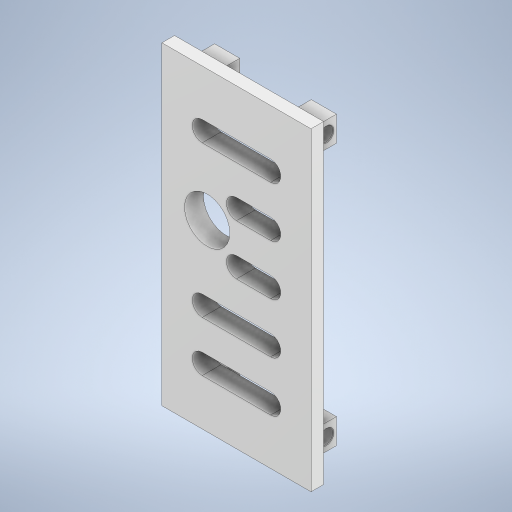
# Autodesk Inventor part: SENSOR_TOP
Saved by Autodesk Inventor 2023 (Build 270158000, 158)
## iProperties
Created: 2023-03-28
Part Number: SENSOR_TOP
Material: PC/ABS Plastic
Document SubType Name: Modeling
Designer: catsm
Density: 0.357273 g/cm^3
Appearance: Smooth - White
Author: catsm
Autodesk Inventor part; units mm, degrees
ref_plane "YZ Plane" through (0, 0, 0) normal (1, 0, 0) x (0, 1, 0)
ref_plane "XZ Plane" through (0, 0, 0) normal (0, 1, 0) x (-1, 0, 0)
ref_plane "XY Plane" through (0, 0, 0) normal (0, 0, 1) x (1, 0, 0)
sketch "Sketch1" plane through (0, 0, 0) normal (0, 0, 1) x (1, 0, 0)
  line L0 (-18.7833, 39.6114) -> (-18.7833, -39.6114) projected
  line L1 (-18.7833, -39.6114) -> (18.7833, -39.6114) projected
  line L2 (18.7833, -39.6114) -> (18.7833, 39.6114) projected
  line L3 (18.7833, 39.6114) -> (-18.7833, 39.6114) projected
  line L4 (-15.6083, 36.4364) -> (15.6083, 36.4364) projected
  line L5 (15.6083, 36.4364) -> (15.6083, -36.4364) projected
  line L6 (15.6083, -36.4364) -> (-15.6083, -36.4364) projected
  line L7 (-15.6083, -36.4364) -> (-15.6083, 36.4364) projected
  point P0 (0, 0)
extrude "Extrusion1" add sketch "Sketch1" along normal blind 3.175 contours L3 L2 L1 L0 | L4 L5 L6 L7
sketch "Sketch2" plane through (0, 0, 0) normal (0, 0, -1) x (-1, 0, 0)
  line L0 (-15.6083, -36.4364) -> (15.6083, -36.4364) projected
  line L1 (-15.6083, 36.4364) -> (-15.6083, -36.4364) projected
  line L2 (15.6083, 36.4364) -> (-15.6083, 36.4364) projected
  line L3 (15.6083, -36.4364) -> (15.6083, 36.4364) projected
  line L4 (-15.3543, 36.1824) -> (-15.3543, -36.1824)
  line L5 (-15.3543, -36.1824) -> (15.3543, -36.1824)
  line L6 (15.3543, -36.1824) -> (15.3543, 36.1824)
  line L7 (15.3543, 36.1824) -> (-15.3543, 36.1824)
  point P0 (0, 0)
  dimension "d2" = 0.254
  constraints: 8 end point, 3 other
  measures "d2" distance between parallel lines of L2 L7
extrude "Extrusion2" add sketch "Sketch2" along normal blind 1.5875 contours L7 L6 L5 L4
sketch "Sketch3" plane through (0, 0, -1.5875) normal (0, 0, -1) x (-1, 0, 0)
  line L0 (-15.3543, 36.1824) -> (-15.3543, -36.1824) projected
  line L1 (-15.3543, 36.1824) -> (-9.0043, 36.1824)
  line L2 (-9.0043, 36.1824) -> (-9.0043, 29.8324)
  line L3 (-9.0043, 29.8324) -> (-15.3543, 29.8324)
  line L4 (-15.3543, 29.8324) -> (-15.3543, 36.1824)
  line L5 (15.3543, 36.1824) -> (-15.3543, 36.1824) projected
  line L6 (15.3543, 36.1824) -> (9.0043, 36.1824)
  line L7 (9.0043, 36.1824) -> (9.0043, 29.8324)
  line L8 (9.0043, 29.8324) -> (15.3543, 29.8324)
  line L9 (15.3543, 29.8324) -> (15.3543, 36.1824)
  line L10 (-15.3543, -36.1824) -> (15.3543, -36.1824) projected
  line L11 (-15.3543, -36.1824) -> (-9.0043, -36.1824)
  line L12 (-9.0043, -36.1824) -> (-9.0043, -29.8324)
  line L13 (-9.0043, -29.8324) -> (-15.3543, -29.8324)
  line L14 (-15.3543, -29.8324) -> (-15.3543, -36.1824)
  line L15 (15.3543, 36.1824) -> (15.3543, -36.1824) projected
  line L16 (15.3543, -36.1824) -> (9.0043, -36.1824)
  line L17 (9.0043, -36.1824) -> (9.0043, -29.8324)
  line L18 (9.0043, -29.8324) -> (15.3543, -29.8324)
  line L19 (15.3543, -29.8324) -> (15.3543, -36.1824)
  point P0 (0, 0)
  dimension "d5" = 6.35
  dimension "d6" = 6.35
  dimension "d7" = 6.35
  dimension "d8" = 6.35
  dimension "d9" = 6.35
  dimension "d10" = 6.35
  dimension "d11" = 6.35
  dimension "d12" = 6.35
  constraints: 32 end point, 8 parallel, 4 horizontal, 4 perpendicular
  measures "d5" distance of L2.end L3.end
  measures "d6" distance of L1.end L2.end
  measures "d7" distance of L8.end L7.end
  measures "d8" distance of L7.end L6.end
  measures "d9" distance of L13.end L12.end
  measures "d10" distance of L12.end L11.end
  measures "d11" distance of L17.end L18.end
  measures "d12" distance of L16.end L17.end
extrude "Extrusion3" add sketch "Sketch3" along normal blind 5.08 contours L1 L2 L3 L0 | L13 L12 L10 L0 | L5 L9 L8 L7 | L17 L18 L15 L10
sketch "Sketch4" plane through (15.3543, -36.1824, 0) normal (1, 0, 0) x (0, 0, -1)
  line L0 (6.6675, 66.0147) -> (6.6675, 72.3647) projected
  line L1 (0, 72.3647) -> (0, 0) projected
  line L2 (6.6675, 0) -> (6.6675, 6.35) projected
  line L3 (1.5875, 66.0147) -> (1.5875, 6.35) projected
  line L4 (0, 72.3647) -> (6.6675, 72.3647) projected
  line L5 (1.5875, 6.35) -> (6.6675, 6.35) projected
  line L6 (6.6675, 6.35) -> (6.6675, 0) projected
  line L7 (1.5875, 6.35) -> (6.6675, 0)
  line L8 (1.5875, 66.0147) -> (6.6675, 72.3647)
  point P0 (0, 36.1824)
  point P1 (4.1275, 3.175)
  point P2 (4.1275, 69.1897)
  point P3 (4.1275, 3.175)
  point P4 (4.1275, 69.1897)
  constraints: 4 end point, 2 coincident, 2 midpoint
sketch "Sketch5" plane through (-15.3543, -36.1824, 0) normal (-1, 0, 0) x (0, 0, 1)
  point P0 (0, 36.1824)
  point P1 (-4.1275, 69.1897)
  point P2 (-4.1275, 3.175)
hole "Hole1" at (15.3543, 33.0074, -4.1275) at (15.3543, -33.0074, -4.1275) direction (-1, 0, 0) diameter 3.556 depth 5.842 countersink diameter 3.81 countersink angle 82
hole "Hole2" at (-15.3543, 33.0074, -4.1275) at (-15.3543, -33.0074, -4.1275) direction (1, 0, 0) diameter 3.556 depth 5.842 countersink diameter 3.81 countersink angle 82
sketch "Sketch6" plane through (0, 0, 3.175) normal (0, 0, 1) x (1, 0, 0)
  line L0 (-8.6233, 0) -> (8.6233, 0) construction
  line L1 (-8.6233, 2.54) -> (8.6233, 2.54)
  line L2 (8.6233, -2.54) -> (-8.6233, -2.54)
  arc A0 (-8.6233, 2.54) -> (-8.6233, -2.54) centre (-8.6233, 0) ccw
  arc A1 (8.6233, -2.54) -> (8.6233, 2.54) centre (8.6233, 0) ccw
  line L3 (-18.7833, 39.6114) -> (-18.7833, -39.6114) projected
  line L4 (18.7833, -39.6114) -> (18.7833, 39.6114) projected
  line L5 (-18.7833, -39.6114) -> (18.7833, -39.6114) projected
  arc A2 (8.6233, 10.16) -> (8.6233, 15.24) centre (8.6233, 12.7) ccw
  line L6 (-8.6233, 15.24) -> (8.6233, 15.24)
  line L7 (8.6233, 10.16) -> (-8.6233, 10.16)
  arc A3 (-8.6233, 15.24) -> (-8.6233, 10.16) centre (-8.6233, 12.7) ccw
  arc A4 (8.6233, 22.86) -> (8.6233, 27.94) centre (8.6233, 25.4) ccw
  line L8 (-8.6233, 27.94) -> (8.6233, 27.94)
  line L9 (8.6233, 22.86) -> (-8.6233, 22.86)
  arc A5 (-8.6233, 27.94) -> (-8.6233, 22.86) centre (-8.6233, 25.4) ccw
  arc A6 (8.6233, -15.24) -> (8.6233, -10.16) centre (8.6233, -12.7) ccw
  line L10 (-8.6233, -10.16) -> (8.6233, -10.16)
  line L11 (8.6233, -15.24) -> (-8.6233, -15.24)
  arc A7 (-8.6233, -10.16) -> (-8.6233, -15.24) centre (-8.6233, -12.7) ccw
  arc A8 (8.6233, -2.54) -> (8.6233, 2.54) centre (8.6233, 0) ccw
  line L12 (-8.6233, 2.54) -> (8.6233, 2.54)
  line L13 (8.6233, -2.54) -> (-8.6233, -2.54)
  arc A9 (-8.6233, 2.54) -> (-8.6233, -2.54) centre (-8.6233, 0) ccw
  arc A10 (8.6233, 10.16) -> (8.6233, 15.24) centre (8.6233, 12.7) ccw
  line L14 (-8.6233, 15.24) -> (8.6233, 15.24)
  line L15 (8.6233, 10.16) -> (-8.6233, 10.16)
  arc A11 (-8.6233, 15.24) -> (-8.6233, 10.16) centre (-8.6233, 12.7) ccw
  arc A12 (8.6233, -27.94) -> (8.6233, -22.86) centre (8.6233, -25.4) ccw
  line L16 (-8.6233, -22.86) -> (8.6233, -22.86)
  line L17 (8.6233, -27.94) -> (-8.6233, -27.94)
  arc A13 (-8.6233, -22.86) -> (-8.6233, -27.94) centre (-8.6233, -25.4) ccw
  arc A14 (8.6233, -15.24) -> (8.6233, -10.16) centre (8.6233, -12.7) ccw
  line L18 (-8.6233, -10.16) -> (8.6233, -10.16)
  line L19 (8.6233, -15.24) -> (-8.6233, -15.24)
  arc A15 (-8.6233, -10.16) -> (-8.6233, -15.24) centre (-8.6233, -12.7) ccw
  arc A16 (8.6233, -2.54) -> (8.6233, 2.54) centre (8.6233, 0) ccw
  line L20 (-8.6233, 2.54) -> (8.6233, 2.54)
  line L21 (8.6233, -2.54) -> (-8.6233, -2.54)
  arc A17 (-8.6233, 2.54) -> (-8.6233, -2.54) centre (-8.6233, 0) ccw
  circle A18 centre (0, 12.7) radius 2.54
  circle A19 centre (0, 0) radius 2.54
  point P0 (0, 0)
  point P1 (0, 10.16)
  point P2 (0, 15.24)
  point P3 (0, 2.54)
  point P4 (0, -2.54)
  dimension "d29" = 10.16
  dimension "d30" = 10.16
  dimension "d31" = 2.54
  dimension "d35" = 12.7
  dimension "d38" = 12.7
  constraints: 40 end point, 36 point on circle, 20 centre point, 4 tangent, 2 vertical, 1 coincident, 1 horizontal, 1 midpoint, 1 parallel, 80 other
  measures "d29" distance from line of L3 L0.start
  measures "d30" distance from line of L4 L0.end
  measures "d31" radius of A1
  measures "d35" distance of L0.end A2.centre
  measures "d38" distance of L0.end A6.centre
extrude "Extrusion4" cut sketch "Sketch6" against normal up to surface (4.7625 mm away) contours L1 A1 L2 A19 | A19 | L7 A18 L6 A2 | A18 | L9 A5 L8 A4 | L11 A7 L10 A6 | L17 A13 L16 A12
sketch "Sketch7" plane through (0, 0, 3.175) normal (0, 0, 1) x (1, 0, 0)
  circle A0 centre (-7.3787, 6.5914) radius 5.715
  line L0 (18.7833, 39.6114) -> (-18.7833, 39.6114) projected
  line L1 (-18.7833, 39.6114) -> (-18.7833, -39.6114) projected
  line L2 (18.7833, -39.6114) -> (18.7833, 39.6114) projected
  point P0 (0, 0)
  dimension "d43" = 11.43
  dimension "d44" = 33.02
  dimension "d46" = 26.162
  constraints: 1 centre point
  measures "d43" diameter of A0
  measures "d44" distance from line of L0 A0.centre
  measures "d46" distance from line of L2 A0.centre
extrude "Extrusion5" cut sketch "Sketch7" against normal up to surface (4.7625 mm away)
body "Solid1"
